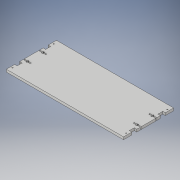
# Autodesk Inventor part: wall-front
Saved by Autodesk Inventor 2017 (Build 210142000, 142)
## iProperties
Created: 2017-02-28
Part Number: wall-front
Material: Generic
Document SubType Name: Modeling
Designer: John
Density: 1 g/cm^3
Appearance: Default
Author: John
Autodesk Inventor part; units mm, degrees
ref_plane "YZ Plane" through (0, 0, 0) normal (1, 0, 0) x (0, 1, 0)
ref_plane "XZ Plane" through (0, 0, 0) normal (0, 1, 0) x (-1, 0, 0)
ref_plane "XY Plane" through (0, 0, 0) normal (0, 0, 1) x (1, 0, 0)
sketch "Sketch1" plane through (0, 0, 0) normal (0, 1, 0) x (-1, 0, 0)
  line L0 (0, 0) -> (-283, 0)
  line L1 (-283, -121) -> (0, -121)
  line L2 (-283, -101) -> (-277, -101)
  line L3 (-277, -101) -> (-277, -89)
  line L4 (-277, -89) -> (-283, -89)
  line L5 (-283, -89) -> (-283, -101) construction
  line L6 (-283, -20) -> (-277, -20)
  line L7 (-277, -20) -> (-277, -32)
  line L8 (-277, -32) -> (-283, -32)
  line L9 (-283, -32) -> (-283, -20) construction
  line L10 (-141.5, 0) -> (-141.5, -121) construction
  line L11 (-283, -20) -> (-283, 0)
  line L12 (-283, -32) -> (-283, -40.5)
  line L13 (-283, -101) -> (-283, -121)
  circle A0 centre (-278.75, -10.75) radius 1.25
  line L14 (-278.75, -10.75) -> (-278.75, -20) construction
  circle A1 centre (-278.75, -110.25) radius 1.25
  line L15 (-283, -80.5) -> (-275, -80.5)
  line L16 (-266, -80.5) -> (-266, -78)
  line L17 (-266, -78) -> (-272.7, -78)
  line L18 (-283, -40.5) -> (-275, -40.5)
  line L19 (-266, -40.5) -> (-266, -43)
  line L20 (-266, -43) -> (-272.7, -43)
  line L21 (-283, -80.5) -> (-283, -89)
  line L22 (-283, -78) -> (-283, -80.5) construction
  line L23 (-283, -43) -> (-283, -78)
  line L24 (-283, -40.5) -> (-283, -43) construction
  line L25 (-272.7, -44.45) -> (-275, -44.45)
  line L26 (-275, -44.45) -> (-275, -43)
  line L27 (-275, -39.05) -> (-272.7, -39.05)
  line L28 (-272.7, -39.05) -> (-272.7, -40.5)
  line L29 (-275, -43) -> (-275, -40.5) construction
  line L30 (-275, -40.5) -> (-275, -39.05)
  line L31 (-272.7, -43) -> (-272.7, -44.45)
  line L32 (-272.7, -40.5) -> (-272.7, -43) construction
  line L33 (-272.7, -40.5) -> (-266, -40.5)
  line L34 (-275, -40.5) -> (-272.7, -40.5) construction
  line L35 (-272.7, -43) -> (-275, -43) construction
  line L36 (-275, -43) -> (-283, -43)
  line L37 (-272.7, -81.95) -> (-275, -81.95)
  line L38 (-275, -81.95) -> (-275, -80.5)
  line L39 (-275, -76.55) -> (-272.7, -76.55)
  line L40 (-272.7, -76.55) -> (-272.7, -78)
  line L41 (-272.7, -80.5) -> (-272.7, -81.95)
  line L42 (-272.7, -78) -> (-272.7, -80.5) construction
  line L43 (-275, -80.5) -> (-275, -78) construction
  line L44 (-275, -78) -> (-275, -76.55)
  line L45 (-275, -80.5) -> (-272.7, -80.5) construction
  line L46 (-272.7, -80.5) -> (-266, -80.5)
  line L47 (-272.7, -78) -> (-275, -78) construction
  line L48 (-275, -78) -> (-283, -78)
  line L49 (0, -101) -> (-6, -101)
  line L50 (-6, -101) -> (-6, -89)
  line L51 (-6, -89) -> (0, -89)
  line L52 (0, -89) -> (0, -101) construction
  line L53 (0, -20) -> (-6, -20)
  line L54 (-6, -20) -> (-6, -32)
  line L55 (-6, -32) -> (0, -32)
  line L56 (0, -32) -> (0, -20) construction
  line L57 (0, -20) -> (0, 0)
  line L58 (0, -32) -> (0, -40.5)
  line L59 (0, -101) -> (0, -121)
  circle A2 centre (-4.25, -10.75) radius 1.25
  line L60 (-4.25, -10.75) -> (-4.25, -20) construction
  circle A3 centre (-4.25, -110.25) radius 1.25
  line L61 (0, -80.5) -> (-8, -80.5)
  line L62 (-17, -80.5) -> (-17, -78)
  line L63 (-17, -78) -> (-10.3, -78)
  line L64 (0, -40.5) -> (-8, -40.5)
  line L65 (-17, -40.5) -> (-17, -43)
  line L66 (-17, -43) -> (-10.3, -43)
  line L67 (0, -80.5) -> (0, -89)
  line L68 (0, -78) -> (0, -80.5) construction
  line L69 (0, -43) -> (0, -78)
  line L70 (0, -40.5) -> (0, -43) construction
  line L71 (-10.3, -44.45) -> (-8, -44.45)
  line L72 (-8, -44.45) -> (-8, -43)
  line L73 (-8, -39.05) -> (-10.3, -39.05)
  line L74 (-10.3, -39.05) -> (-10.3, -40.5)
  line L75 (-8, -43) -> (-8, -40.5) construction
  line L76 (-8, -40.5) -> (-8, -39.05)
  line L77 (-10.3, -43) -> (-10.3, -44.45)
  line L78 (-10.3, -40.5) -> (-10.3, -43) construction
  line L79 (-10.3, -40.5) -> (-17, -40.5)
  line L80 (-8, -40.5) -> (-10.3, -40.5) construction
  line L81 (-10.3, -43) -> (-8, -43) construction
  line L82 (-8, -43) -> (0, -43)
  line L83 (-10.3, -81.95) -> (-8, -81.95)
  line L84 (-8, -81.95) -> (-8, -80.5)
  line L85 (-8, -76.55) -> (-10.3, -76.55)
  line L86 (-10.3, -76.55) -> (-10.3, -78)
  line L87 (-10.3, -80.5) -> (-10.3, -81.95)
  line L88 (-10.3, -78) -> (-10.3, -80.5) construction
  line L89 (-8, -80.5) -> (-8, -78) construction
  line L90 (-8, -78) -> (-8, -76.55)
  line L91 (-8, -80.5) -> (-10.3, -80.5) construction
  line L92 (-10.3, -80.5) -> (-17, -80.5)
  line L93 (-10.3, -78) -> (-8, -78) construction
  line L94 (-8, -78) -> (0, -78)
  dimension "d0" = 283
  dimension "d1" = 121
  dimension "d20" = 6
  dimension "d21" = 12
  dimension "d22" = 12
  dimension "d26" = 57
  dimension "d27" = 2.5
  dimension "d28" = 4.25
  dimension "d29" = 9.25
  dimension "d30" = 2.5
  dimension "d31" = 4.25
  dimension "d32" = 9.25
  dimension "d33" = 17
  dimension "d34" = 2.5
  dimension "d35" = 17
  dimension "d36" = 2.5
  dimension "d37" = 8.5
  dimension "d39" = 20
  dimension "d40" = 2.3
  dimension "d41" = 5.4
  dimension "d42" = 2.3
  dimension "d43" = 5.4
  dimension "d44" = 8
  dimension "d45" = 8
  constraints: 190 end point, 44 parallel, 35 symmetric about line, 15 perpendicular, 13 collinear, 11 horizontal, 10 point on line, 4 centre point, 2 midpoint, 1 vertical, 2 other
  measures "d0" distance of L1.end L1.start
  measures "d1" distance of L0.end L1.start
  measures "d20" distance of L4.end L3.end
  measures "d21" distance of L3.end L2.end
  measures "d22" distance of L6.end L7.end
  measures "d26" distance of L8.end L4.end
  measures "d27" diameter of A0
  measures "d28" distance from line of L11 L14.start
  measures "d29" distance of L14.start L14.end
  measures "d30" diameter of A1
  measures "d31" distance from line of L13 A1.centre
  measures "d32" distance from line of L2 A1.centre
  measures "d33" distance of L22.start L16.end
  measures "d34" distance of L16.end L16.start
  measures "d35" distance of L19.end L23.start
  measures "d36" distance of L19.start L19.end
  measures "d37" distance of L15.start L4.end
  measures "d39" distance between parallel lines of L0 L6
  measures "d40" distance of L27.start L27.end
  measures "d41" distance of L25.end L27.start
  measures "d42" distance of L39.start L39.end
  measures "d43" distance of L37.end L39.start
  measures "d44" distance between parallel lines of L21 L38
  measures "d45" distance between parallel lines of L23 L26
extrude "Extrusion2" add sketch "Sketch1" along normal blind 6
equation "\"d22\" = d21"
equation "\"d30\" = d27"
equation "\"d31\" = d28"
equation "\"d32\" = d29"
equation "\"d33\" = d35"
equation "\"d34\" = d36"
equation "\"d42\" = d40"
equation "\"d43\" = d41"
equation "\"d44\" = d45"
body "Solid2"
